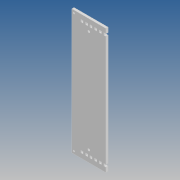
# Autodesk Inventor part: KB33-046-004-005 - Лицевая наклонная пластина
Saved by Autodesk Inventor 2020 (Build 240168000, 168)
## iProperties
Created: 2021-06-25
Part Number: KB33-046-004-005 - Лицевая наклонная пластина
Material: Типовые
Document SubType Name: Modeling
Designer: Петров Иван
Mass: 51.635 g
Surface Area: 289.294 cm^2
Volume: 51.635 cm^3
Density: 1 g/cm^3
Appearance: По умолчанию
Author: Петров Иван
Autodesk Inventor part; units mm, degrees
ref_plane "YZ Plane" through (0, 0, 0) normal (1, 0, 0) x (0, 1, 0)
ref_plane "XZ Plane" through (0, 0, 0) normal (0, 1, 0) x (-1, 0, 0)
ref_plane "XY Plane" through (0, 0, 0) normal (0, 0, 1) x (1, 0, 0)
sketch "Эскиз1" plane through (0, 0, 0) normal (0, 0, 1) x (1, 0, 0)
  circle A0 centre (3.6373, -187.3954) radius 1.5 projected
  circle A1 centre (3.6373, 22.3954) radius 1.5 projected
  line L0 (0, 27) -> (60, 27)
  line L1 (60, 27) -> (60, -190.5454)
  line L2 (60, -190.5454) -> (0, -190.5454)
  line L3 (0, -190.5454) -> (0, 27)
  point P0 (0, 0)
  point P1 (0, -190.5454)
  dimension "d0" = 60
  constraints: 8 end point, 2 parallel, 1 horizontal, 1 perpendicular, 2 other
  measures "d0" distance of L1.end L2.end
extrude "Выдавливание1" add sketch "Эскиз1" along normal blind 4
thicken "Толщина1" operation add thickness 1.455 both sides no extend neighbours yes toward (0, -1, 0) faces at (20, -190.5454, 2.6667)
sketch "Эскиз2" plane through (0, 0, 4) normal (0, 0, 1) x (1, 0, 0)
  line L0 (60, 19) -> (56, 19)
  line L1 (56, 19) -> (56, 15)
  line L2 (56, 15) -> (60, 15)
  line L3 (60, 15) -> (60, 19)
  line L4 (60, -192.0004) -> (60, 27) projected
  line L5 (60, 27) -> (0, 27) projected
  point P0 (0, 0)
  dimension "d5" = 4
  dimension "d6" = 4
  dimension "d7" = 8
  constraints: 8 end point, 2 parallel, 1 horizontal, 1 perpendicular, 1 point on line
  measures "d5" distance of L2.end L1.end
  measures "d6" distance of L1.end L0.end
  measures "d7" distance between parallel lines of L5 L0
extrude "Выдавливание2" cut sketch "Эскиз2" against normal blind 10
pattern_linear "Прямоуг.массив1" count 6 spacing 8 along (-1, 0, 0) of "Выдавливание2"
ref_plane "РабПлоскость1" through (0, -82.5002, 4) normal (0, 1, 0) x (1, 0, 0)
mirror "Зеркальное отражение1" about plane through (0, -82.5002, 4) normal (0, 1, 0) of "Выдавливание2", "Прямоуг.массив1"
sketch "Эскиз3" plane through (0, 0, 4) normal (0, 0, 1) x (1, 0, 0)
  circle A0 centre (30, 7.5) radius 2
  circle A1 centre (30, -172.5) radius 2
  point P0 (0, 0)
  point P1 (0, 0)
  constraints: 2 centre point
extrude "Выдавливание3" cut sketch "Эскиз3" against normal blind 10
